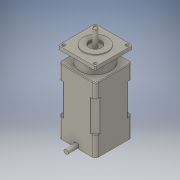
# Autodesk Inventor part: ElectrocraftE3266
Saved by Autodesk Inventor 2019 (Build 230136000, 136)
## iProperties
Created: 2019-05-08
Part Number: ElectrocraftE3266
Material: Steel, High Strength, Low Alloy
Document SubType Name: Modeling
Designer: Jorian Bruslind
Density: 7.85 g/cm^3
Appearance: Steel - Cast
Author: Jorian Bruslind
Autodesk Inventor part; units mm, degrees
ref_plane "YZ Plane" through (0, 0, 0) normal (1, 0, 0) x (0, 1, 0)
ref_plane "XZ Plane" through (0, 0, 0) normal (0, 1, 0) x (-1, 0, 0)
sketch "Sketch1" plane through (0, 0, 0) normal (0, 1, 0) x (-1, 0, 0)
  line L0 (0, 0) -> (57.5, 0)
  line L1 (57.5, 0) -> (57.5, -57.5)
  line L2 (57.5, -57.5) -> (0, -57.5)
  line L3 (0, -57.5) -> (0, 0)
  dimension "d0" = 57.5
  dimension "d1" = 57.5
  constraints: 8 end point, 2 parallel, 1 horizontal, 1 perpendicular
  measures "d0" distance of L1.end L2.end
  measures "d1" distance of L0.end L1.end
extrude "Extrusion1" add sketch "Sketch1" along normal blind 100.75
sketch "Sketch3" plane through (0, 100.75, 0) normal (0, 1, 0) x (1, 0, 0)
  circle A0 centre (-28.75, 28.75) radius 24
  line L0 (0, 0) -> (0, 57.5) projected
  line L1 (-57.5, 0) -> (0, 0) projected
  dimension "d8" = 48
  dimension "d9" = 28.75
  dimension "d10" = 28.75
  constraints: 1 centre point
  measures "d8" diameter of A0
  measures "d9" distance from line of L0 A0.centre
  measures "d10" distance from line of L1 A0.centre
extrude "Extrusion2" add sketch "Sketch3" along normal blind 17.5
sketch "Sketch4" plane through (-28.75, 118.25, -28.75) normal (0, 1, 0) x (1, 0, 0)
  line L0 (28.75, 28.75) -> (-28.75, 28.75) projected
  line L1 (-28.75, -28.75) -> (28.75, -28.75) projected
  line L2 (28.75, 28.75) -> (-28.75, 28.75)
  line L3 (-28.75, 28.75) -> (-28.75, -28.75)
  line L4 (-28.75, -28.75) -> (28.75, -28.75)
  line L5 (28.75, -28.75) -> (28.75, 28.75)
  constraints: 8 end point, 2 parallel, 1 horizontal, 1 perpendicular
extrude "Extrusion3" add sketch "Sketch4" along normal blind 5.25
sketch "Sketch5" plane through (-28.75, 123.5, -28.75) normal (0, 1, 0) x (1, 0, 0)
  circle A0 centre (0, 0) radius 19
  line L0 (-28.75, 28.75) -> (-28.75, -28.75) projected
  line L1 (28.75, 28.75) -> (-28.75, 28.75) projected
  point P0 (28.75, -28.75)
  dimension "d15" = 38
  dimension "d16" = 28.75
  dimension "d17" = 28.75
  constraints: 1 centre point
  measures "d15" diameter of A0
  measures "d16" distance from line of L0 A0.centre
  measures "d17" distance from line of L1 A0.centre
extrude "Extrusion4" add sketch "Sketch5" along normal blind 1.3
sketch "Sketch6" plane through (-28.75, 124.8, -28.75) normal (0, 1, 0) x (1, 0, 0)
  circle A0 centre (0, 0) radius 9.5
  line L0 (28.75, -28.75) -> (28.75, 28.75) projected
  line L1 (-28.75, -28.75) -> (28.75, -28.75) projected
  dimension "d20" = 19
  dimension "d21" = 28.75
  dimension "d22" = 28.75
  constraints: 1 centre point
  measures "d20" diameter of A0
  measures "d21" distance from line of L0 A0.centre
  measures "d22" distance from line of L1 A0.centre
extrude "Extrusion5" cut sketch "Sketch6" against normal blind 3.61
sketch "Sketch7" plane through (-28.75, 121.19, -28.75) normal (0, 1, 0) x (1, 0, 0)
  circle A0 centre (0, 0) radius 9.5 projected
  circle A1 centre (0, 0) radius 3.25
  point P0 (28.75, -28.75)
  dimension "d25" = 6.5
  constraints: 1 centre point, 1 coincident
  measures "d25" diameter of A1
extrude "Extrusion6" add sketch "Sketch7" along normal blind 25 contours A1
sketch "Sketch8" plane through (-28.75, 123.5, -28.75) normal (0, 1, 0) x (1, 0, 0)
  circle A0 centre (24.46, -24.46) radius 2.5
  line L0 (-28.75, -28.75) -> (28.75, -28.75) projected
  line L1 (28.75, -28.75) -> (28.75, 28.75) projected
  circle A1 centre (24.46, 24.54) radius 2.5
  circle A2 centre (-24.54, -24.46) radius 2.5
  circle A3 centre (-24.54, 24.54) radius 2.5
  dimension "d28" = 5
  dimension "d29" = 4.29
  dimension "d30" = 4.29
  dimension "d33" = 49
  dimension "d36" = 49
  constraints: 4 centre point, 1 horizontal, 1 vertical, 6 other
  measures "d28" diameter of A0
  measures "d29" distance from line of L0 A0.centre
  measures "d30" distance from line of L1 A0.centre
  measures "d33" distance of A0.centre A1.centre
  measures "d36" distance of A0.centre A2.centre
extrude "Extrusion7" cut sketch "Sketch8" against normal blind 5.25
ref_plane "Work Plane1" through (-57.5, 0, -57.5) normal (-0.7071068, 0, -0.7071068) x (0, 1, 0)
sketch "Sketch9" plane through (-57.5, 0, -57.5) normal (-0.7071068, 0, -0.7071068) x (0, 1, 0)
  line L0 (0, 0) -> (100.75, 0) projected
  line L1 (100.75, 0) -> (77.75, 0)
  line L2 (77.75, 0) -> (30.75, 0)
  line L3 (77.75, 9.5) -> (30.75, 9.5)
  line L4 (30.75, 9.5) -> (30.75, -9.5)
  line L5 (30.75, -9.5) -> (77.75, -9.5)
  line L6 (77.75, -9.5) -> (77.75, 9.5)
  line L7 (77.75, 9.5) -> (30.75, -9.5) construction
  line L8 (30.75, 9.5) -> (77.75, -9.5) construction
  point P0 (54.25, 0)
  dimension "d42" = 23
  dimension "d43" = 47
  dimension "d44" = 47
  dimension "d45" = 19
  constraints: 16 end point, 3 midpoint, 2 parallel, 2 point on line, 1 horizontal, 1 perpendicular
  measures "d42" distance of L0.end L1.end
  measures "d43" distance of L1.end L2.end
  measures "d44" distance of L5.end L4.end
  measures "d45" distance of L4.end L3.end
extrude "Extrusion8" cut sketch "Sketch9" against normal blind 5.5
pattern_circular "Circular Pattern1" count 4 over 360 about axis through (-28.75, 124.8, -28.75) along (0, -1, 0) of "Extrusion8"
sketch "Sketch10" plane through (0, 0, 0) normal (0, -1, 0) x (1, 0, 0)
  circle A0 centre (-28.75, -28.75) radius 3.25 projected
  circle A1 centre (-28.75, -28.75) radius 20.5
  line L0 (0, 0) -> (0, -57.5) projected
  line L1 (0, -57.5) -> (-15.315, -42.185)
  circle A2 centre (-28.75, -28.75) radius 19 projected
  line L2 (0, -57.5) -> (21.6586, -57.5) construction
  line L3 (-14.2543, -43.2457) -> (-10.7612, -46.7388)
  line L4 (-14.2543, -43.2457) -> (-16.7292, -45.7206)
  line L5 (-14.2543, -43.2457) -> (-10.7543, -43.2457) construction
  line L6 (-14.2543, -43.2457) -> (-11.7794, -40.7708)
  line L7 (-11.4259, -41.1244) -> (-6.8297, -45.7206)
  line L8 (-6.8297, -45.7206) -> (-11.7794, -50.6703)
  line L9 (-11.7794, -50.6703) -> (-16.7292, -45.7206)
  line L10 (-16.7292, -45.7206) -> (-16.3756, -46.0741)
  spline S0 degree 2 poles (-14.2543, -48.1954) (-16.074, -45.3459) (-17.7898, -46.0741) knots 0 0 0 1 1 1
  line L11 (-28.75, -28.75) -> (-43.2457, -43.2457)
  spline S1 degree 2 poles (-9.3046, -43.2457) (-12.1541, -41.426) (-11.4259, -39.7102) knots 0 0 0 1 1 1
  line L12 (-43.2457, -14.2543) -> (-45.7206, -16.7292)
  line L13 (-43.2457, -14.2543) -> (-40.7708, -11.7794)
  line L14 (-41.1244, -11.4259) -> (-45.7206, -6.8297)
  line L15 (-45.7206, -6.8297) -> (-50.6703, -11.7794)
  line L16 (-50.6703, -11.7794) -> (-45.7206, -16.7292)
  spline S2 degree 2 poles (-43.4225, -9.1278) (-41.4383, -12.1839) (-39.7102, -11.4259) knots 0 0 0 1 1 1
  spline S3 degree 2 poles (-48.1954, -14.2543) (-45.4581, -16.0928) (-45.9784, -17.64) knots 0 0 0 1 1 1
  point P0 (-46.0741, -16.3756)
  dimension "d51" = 41
  dimension "d52" = 135
  dimension "d54" = 3.5
  dimension "d55" = 135
  dimension "d56" = 3.5
  dimension "d57" = 7
  dimension "d58" = 7
  dimension "d59" = 0.5
  constraints: 32 end point, 7 symmetric about line, 6 point on circle, 5 point on line, 3 midpoint, 2 equal length, 2 horizontal, 2 perpendicular, 2 tangent, 1 centre point, 1 coincident, 1 parallel, 14 other
  measures "d51" diameter of A1
  measures "d52" angle of L2 L1
  measures "d54" distance of L3.start L4.end
  measures "d55" angle of L4 L5
  measures "d56" distance of L3.start L6.end
  measures "d57" distance of L6.end L7.end
  measures "d58" distance of L7.end L8.end
  measures "d59" distance of L4.end L10.end
extrude "Extrusion9" add sketch "Sketch10" along normal blind 3.85 contours A0 | A1 L1 A2 L11 | A1 L12 L16 S3 L15 L14 S2 | S1 L7 L8 L1 A1 | A1 S3 L16 L12 | L4 L9 S0 A1 | A1 L11 A2 L1 | L1 L8 L9 S0 L4 | A2
sketch "Sketch11" plane through (0, 0, 0) normal (0, -1, 0) x (1, 0, 0)
  arc A0 (-11.4259, -39.7102) -> (-39.7102, -11.4259) centre (-28.75, -28.75) ccw projected
  line L0 (-28.75, -8.25) -> (-28.75, 0)
  line L1 (0, 0) -> (-57.5, 0) projected
  line L2 (-28.75, 0) -> (-57.5, 0)
  line L3 (-25.25, 8.551) -> (-32.25, 8.551)
  line L4 (-32.25, 8.551) -> (-32.25, -8.551)
  line L5 (-32.25, -8.551) -> (-25.25, -8.551)
  line L6 (-25.25, -8.551) -> (-25.25, 8.551)
  line L7 (-25.25, 8.551) -> (-32.25, -8.551) construction
  line L8 (-32.25, 8.551) -> (-25.25, -8.551) construction
  dimension "d62" = 8.25
  dimension "d63" = 7
  constraints: 16 end point, 3 midpoint, 2 horizontal, 2 parallel, 2 point on circle, 1 perpendicular
  measures "d62" distance of L0.start L0.end
  measures "d63" distance of L5.end L4.end
extrude "Extrusion10" cut sketch "Sketch11" against normal blind 6.83
sketch "Sketch12" plane through (-32.25, 0, -8.551) normal (0, 0, 1) x (1, 0, 0)
  circle A0 centre (3.5, 3.33) radius 3.45
  line L0 (7, 6.83) -> (7, 0) projected
  line L1 (0, 6.83) -> (7, 6.83) projected
  point P0 (32.25, 0)
  dimension "d66" = 6.9
  dimension "d67" = 3.5
  dimension "d68" = 3.5
  constraints: 1 centre point
  measures "d66" diameter of A0
  measures "d67" distance from line of L0 A0.centre
  measures "d68" distance from line of L1 A0.centre
extrude "Extrusion11" add sketch "Sketch12" along normal blind 25
sketch "Sketch13" plane through (0, -3.85, 0) normal (0, -1, 0) x (1, 0, 0)
  arc A0 (-11.4259, -39.7102) -> (-39.7102, -11.4259) centre (-28.75, -28.75) ccw projected
  circle A1 centre (-28.75, -28.75) radius 14
  point P0 (0, 0)
  dimension "d71" = 28
  constraints: 1 centre point, 1 coincident
  measures "d71" diameter of A1
extrude "Extrusion12" add sketch "Sketch13" along normal blind 7
fillet "Fillet1" radius 5 8 edges at (0, 89.25, 0) (-57.5, 89.25, 0) (0, 89.25, -57.5) (0, 15.375, -57.5) (0, 15.375, 0) (-57.5, 15.375, 0) (-57.5, 89.25, -57.5) (-57.5, 15.375, -57.5)
fillet "Fillet2" radius 1 8 edges at (-49.719, 54.25, 0) (-57.5, 54.25, -7.781) (-57.5, 54.25, -49.719) (-49.719, 54.25, -57.5) (-7.781, 54.25, -57.5) (0, 54.25, -49.719) (0, 54.25, -7.781) (-7.781, 54.25, 0)
fillet "Fillet3" radius 1 40 edges at (0, 77.75, -7.9881) (0, 77.75, -6.3905) (-6.3905, 77.75, 0) (-7.9881, 77.75, 0) (-1.4645, 77.75, -1.4645) (-1.4645, 77.75, -56.0355) (-6.3905, 77.75, -57.5) (-7.9881, 77.75, -57.5) (0, 77.75, -49.5119) (0, 77.75, -51.1095) (-7.9881, 30.75, 0) (-6.3905, 30.75, 0) (0, 30.75, -7.9881) (0, 30.75, -6.3905) (-1.4645, 30.75, -1.4645) (0, 30.75, -49.5119) (0, 30.75, -51.1095) (-6.3905, 30.75, -57.5) (-7.9881, 30.75, -57.5) (-1.4645, 30.75, -56.0355) (-57.5, 30.75, -7.9881) (-57.5, 30.75, -6.3905) (-49.5119, 30.75, 0) (-51.1095, 30.75, 0) (-56.0355, 30.75, -1.4645) (-49.5119, 77.75, 0) (-51.1095, 77.75, 0) (-57.5, 77.75, -7.9881) (-57.5, 77.75, -6.3905) (-56.0355, 77.75, -1.4645) (-56.0355, 77.75, -56.0355) (-49.5119, 77.75, -57.5) (-51.1095, 77.75, -57.5) (-57.5, 77.75, -51.1095) (-57.5, 77.75, -49.5119) (-56.0355, 30.75, -56.0355) (-49.5119, 30.75, -57.5) (-51.1095, 30.75, -57.5) (-57.5, 30.75, -51.1095) (-57.5, 30.75, -49.5119)
fillet "Fillet4" radius 2 4 edges at (-57.5, 120.875, 0) (-57.5, 120.875, -57.5) (0, 120.875, -57.5) (0, 120.875, 0)
fillet "Fillet5" radius 1 8 edges at (-1.4645, 100.75, -1.4645) (0, 100.75, -28.75) (-1.4645, 100.75, -56.0355) (-28.75, 100.75, -57.5) (-56.0355, 100.75, -56.0355) (-57.5, 100.75, -28.75) (-56.0355, 100.75, -1.4645) (-28.75, 100.75, 0)
fillet "Fillet6" radius 0.5 1 edges at (-32, 146.19, -28.75)
body "Solid1"
